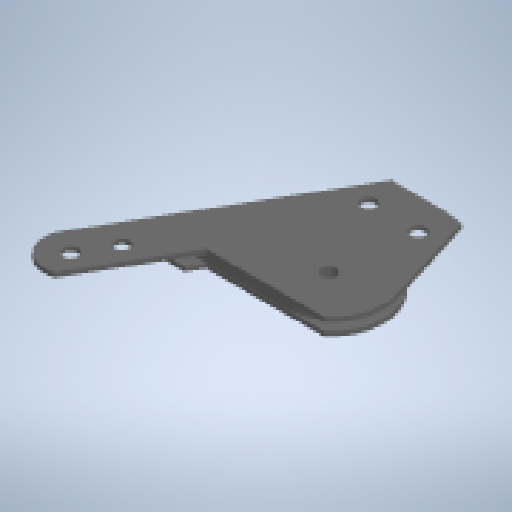
# Autodesk Inventor part: screw_cover_upper
Saved by Autodesk Inventor 2024.1 (Build 281209000, 209)
## iProperties
Created: 2025-01-18
Part Number: screw_cover_upper
Material: 一般
Document SubType Name: Modeling
Designer: hibik
Density: 1 g/cm^3
Appearance: 既定
Author: hibik
Autodesk Inventor part; units mm, degrees
ref_plane "YZ Plane" through (0, 0, 0) normal (1, 0, 0) x (0, 1, 0)
ref_plane "XZ Plane" through (0, 0, 0) normal (0, 1, 0) x (-1, 0, 0)
ref_plane "XY Plane" through (0, 0, 0) normal (0, 0, 1) x (1, 0, 0)
sketch "スケッチ1" plane through (0, 0, 0) normal (0, 1, 0) x (-1, 0, 0)
  circle A0 centre (0, 0) radius 8.9
  line L0 (0, -8.9) -> (63.2748, -8.9)
  line L1 (63.2748, -8.9) -> (63.2748, 8.9)
  line L2 (63.2748, 8.9) -> (0, 8.9)
  line L3 (0, 8.9) -> (0, -8.9)
  circle A1 centre (0, 0) radius 8.4
  line L4 (0, -8.4) -> (63.2748, -8.4)
  line L5 (63.2748, -8.4) -> (63.2748, 8.4)
  line L6 (63.2748, 8.4) -> (0, 8.4)
  line L7 (0, 8.4) -> (0, -8.4)
  point P0 (0, 8.4)
  point P1 (0, 8.9)
  dimension "d0" = 17.8
  dimension "d1" = 16.8
  constraints: 16 end point, 6 horizontal, 4 parallel, 3 coincident, 2 perpendicular, 1 collinear, 6 other
extrude "押し出し1" add sketch "スケッチ1" along normal blind 0.85 contours L3 A1 A0 | L2 L1 L6 A0 | A0 L6 L3 | L3 L4 A0 | A0 L4 L1 L0
sketch "スケッチ2" plane through (0, 0.85, 0) normal (0, 1, 0) x (1, 0, 0)
  circle A0 centre (0, 0) radius 12
  line L0 (0, 12) -> (-63.2748, 12)
  line L1 (-63.2748, 12) -> (-63.2748, -12)
  line L2 (-63.2748, -12) -> (0, -12)
  line L3 (0, -12) -> (0, 12)
  line L4 (-63.2748, 8.9) -> (-63.2748, 8.4) projected
  line L5 (-63.2748, 8.4) -> (0, 8.4) projected
  line L6 (0, -8.4) -> (-63.2748, -8.4) projected
  arc A1 (0, -8.4) -> (0, 8.4) centre (0, 0) ccw projected
  point P0 (0, -12)
  dimension "d4" = 24
  constraints: 8 end point, 3 horizontal, 2 parallel, 1 coincident, 1 collinear, 1 perpendicular, 3 other
extrude "押し出し2" add sketch "スケッチ2" along normal blind 1 contours A0 L3 A1 | L3 L5 A0 | A0 L5 L1 L0 | L2 L1 L6 A0 | A0 L6 L3
mirror "ミラー1" about plane through (-27.1874, 0, 0) normal (0, -1, 0)
sketch "スケッチ3" plane through (0, 1.85, 0) normal (0, 1, 0) x (1, 0, 0)
  line L0 (-10.5885, 24.2158) -> (-40, -26.7265) projected
  line L1 (0, -8.4) -> (-63.2748, -8.4) projected
  line L2 (-63.2748, -8.4) -> (-63.2748, -12) projected
  line L3 (-63.2748, -12) -> (0, -12) projected
  arc A0 (0, -12) -> (0, 12) centre (0, 0) ccw projected
  line L4 (0, 12) -> (-63.2748, 12) projected
  line L5 (-63.2748, 12) -> (-63.2748, 8.4) projected
  line L6 (-63.2748, 8.4) -> (0, 8.4) projected
  arc A1 (0, -8.4) -> (0, 8.4) centre (0, 0) ccw projected
  point P0 (-31.4977, -12)
  point P1 (-29.4192, -8.4)
  point P2 (-19.7197, 8.4)
  point P3 (-17.6412, 12)
extrude "押し出し3" cut sketch "スケッチ3" against normal through all contours L0 L6 L5 L4 | L0 L3 L2 L1
ref_plane "作業平面1" through (0, -0.65, 0) normal (0, 1, 0) x (1, 0, 0)
sketch "スケッチ4" plane through (0, -0.65, 0) normal (0, 1, 0) x (1, 0, 0)
  line L0 (-19.7197, 8.4) -> (0, 8.4) projected
  arc A0 (0, -8.4) -> (0, 8.4) centre (0, 0) ccw projected
  line L1 (0, -8.4) -> (-29.4192, -8.4) projected
  line L2 (-19.7197, 8.4) -> (-29.4192, -8.4)
  circle A1 centre (0, 0) radius 1.6
  dimension "d10" = 3.2
  constraints: 2 coincident, 2 end point, 1 centre point
  measures "d10" diameter of A1
extrude "押し出し4" add sketch "スケッチ4" along normal up to surface (2.5 mm away)
fillet "フィレット1" radius 1 3 edges at (-9.8599, -0.65, -8.4) (8.4, -0.65, 0) (-14.7096, -0.65, 8.4)
sketch "スケッチ5" plane through (0, 1.85, 0) normal (0, 1, 0) x (1, 0, 0)
  circle A0 centre (-27.8315, -17.35) radius 1.6 projected
  circle A1 centre (-8.7282, 17.4379) radius 1.6 projected
  line L0 (0, 12) -> (-17.6412, 12) projected
  line L1 (-17.6412, 12) -> (-10.5885, 24.2158)
  line L2 (-10.5885, 24.2158) -> (0, 24.2158)
  line L3 (-19.3733, 9) -> (-10.5885, 24.2158) projected
  line L4 (0, 12) -> (-17.6412, 12) projected
  circle A2 centre (0, 0) radius 24.2158
  arc A3 (0, -12) -> (0, 12) centre (0, 0) ccw projected
  line L5 (11.4695, 3.5285) -> (5.2849, 23.6321)
  circle A4 centre (1.9592, 17.4379) radius 1.6
  line L6 (-40, -26.7265) -> (-29.7656, -9) projected
  circle A5 centre (-31.9338, -24.4553) radius 1.6 projected
  circle A6 centre (-36, -34.6362) radius 1.6 projected
  circle A7 centre (-27.8315, -17.35) radius 1.6 projected
  line L7 (-17.7656, -9) -> (-29.7656, -9) projected
  line L8 (-40, -26.7265) -> (-29.7656, -9) projected
  line L9 (-40, -50.5) -> (-40, -26.7265) projected
  line L10 (-37.5, -50.5) -> (-40, -50.5) projected
  line L11 (-31, -42.5) -> (-31, -31.9226) projected
  line L12 (-31, -31.9226) -> (-17.7656, -9) projected
  line L13 (-37.5, -50.5) -> (-37.5, -42.5) projected
  line L14 (-37.5, -42.5) -> (-31, -42.5) projected
  circle A8 centre (-31.9338, -24.4553) radius 5.85
  point P0 (-20.2427, -13.2905)
  point P1 (-22.4812, -9)
  point P2 (-12.6465, 20.6512)
  point P3 (-37, -21.5303)
  point P4 (-29.8432, -29.9191)
  dimension "d14" = 15
  dimension "d15" = 3.2
  dimension "d16" = 5
  constraints: 6 end point, 3 centre point, 3 point on circle, 3 tangent, 2 coincident, 1 collinear, 1 horizontal alignment, 1 parallel, 1 point on line
  measures "d14" distance from line of L1.end L5
  measures "d15" diameter of A4
  measures "d16" distance from line of L5 A4.centre
extrude "押し出し5" add sketch "スケッチ5" against normal blind 1 contours L0 L1 A2 L5 A3 | L1 L2 A2 | L7 L12 A2 | A2 L12 A8 L6 L7 | L12 A8 picked at (-28.839, -26.2173)
sketch "スケッチ6" plane through (0, 1.85, 0) normal (0, 1, 0) x (1, 0, 0)
  line L0 (-19.4977, -12) -> (0, -12) projected
  line L1 (-19.4977, -12) -> (-17.7656, -9)
  line L2 (-17.7656, -9) -> (7.9373, -9)
  arc A0 (0, -12) -> (0, 12) centre (0, 0) ccw projected
  line L3 (-29.8432, -29.9191) -> (-19.4977, -12) projected
  point P0 (-25.741, -22.8137)
  point P1 (-20.2427, -13.2905)
  point P2 (-31, -31.9226)
  dimension "d19" = 3
  constraints: 4 end point, 1 collinear, 1 parallel, 1 point on circle
  measures "d19" distance between parallel lines of L2 L0
extrude "押し出し6" cut sketch "スケッチ6" against normal through all
